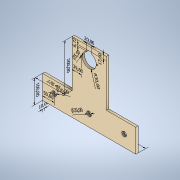
# Autodesk Inventor part: InnenUnten
Saved by Autodesk Inventor 2020.3 (Build 243373010, 373A)
## iProperties
Created: 2021-02-11
Part Number: InnenUnten
Material: Generisch
Document SubType Name: Modeling
Designer: Stefan
Density: 1 g/cm^3
Appearance: Pappel
Author: Stefan
Autodesk Inventor part; units mm, degrees
ref_plane "YZ Plane" through (0, 0, 0) normal (1, 0, 0) x (0, 1, 0)
ref_plane "XZ Plane" through (0, 0, 0) normal (0, 1, 0) x (-1, 0, 0)
ref_plane "XY Plane" through (0, 0, 0) normal (0, 0, 1) x (1, 0, 0)
sketch "Skizze1" plane through (0, 0, 0) normal (0, 0, 1) x (1, 0, 0)
  line L0 (147.1952, 0) -> (147.1952, 200)
  line L1 (147.1952, 200) -> (0, 200)
  line L2 (0, 200) -> (0, 0)
  line L3 (0, 0) -> (-24.1421, 0)
  line L4 (-24.1421, 0) -> (-126.4024, 0)
  line L5 (-126.4024, 0) -> (-126.4024, -100)
  line L6 (-126.4024, -100) -> (273.5976, -100)
  line L7 (273.5976, -100) -> (273.5976, 0)
  line L8 (273.5976, 0) -> (171.3373, 0)
  line L9 (171.3373, 0) -> (147.1952, 0)
  circle A0 centre (223.5976, -50) radius 10
  circle A1 centre (-76.4024, -50) radius 10
  circle A2 centre (73.5976, -50) radius 10
  dimension "d34" = 20
  dimension "d35" = 90
  dimension "d36" = 90
  dimension "d37" = 90
  dimension "d38" = 126.4024
  dimension "d39" = 273.5976
  dimension "d40" = 400
  dimension "d41" = 200
  dimension "d42" = 100
  dimension "d43" = 0
  dimension "d44" = 0
  dimension "d45" = 0
  dimension "d46" = 0
  dimension "d47" = 0
  dimension "d48" = 100
  dimension "d49" = 0
  dimension "d50" = 50
  dimension "d51" = 50
  dimension "d52" = 102.2603
  dimension "d53" = 102.2603
  dimension "d54" = 200
  dimension "d55" = 126.4024
  dimension "d56" = 0
  dimension "d57" = 126.4024
  dimension "d58" = 200
  dimension "d59" = 50
  dimension "d60" = 200
  dimension "d61" = 273.5976
  dimension "d62" = 0
  dimension "d63" = 273.5976
  dimension "d64" = 297.7397
  dimension "d65" = 297.7397
  dimension "d66" = 350
  dimension "d67" = 50
  dimension "d68" = 0
  dimension "d69" = 400
  dimension "d70" = 100
  dimension "d71" = 400
  constraints: 20 end point, 5 parallel, 3 centre point, 2 equal radius, 1 horizontal, 1 vertical
  measures "d34" diameter of A0
  measures "d35" angle of L7 L8
  measures "d36" angle of L7 L3
  measures "d37" angle of L7 L4
  measures "d38" distance between parallel lines of L0 L7
  measures "d39" distance between parallel lines of L2 L7
  measures "d40" distance between parallel lines of L5 L7
  measures "d41" distance between parallel lines of L1 L9
  measures "d42" distance between parallel lines of L6 L9
  measures "d43" distance from line of L7.end L8
  measures "d44" distance from line of L7.end L9
  measures "d45" distance from line of L7.end L3
  measures "d46" distance from line of L7.end L4
  measures "d47" distance from line of L8.start L7
  measures "d48" distance from line of L7.start L8
  measures "d49" distance from line of L6.end L7
  measures "d50" distance from line of A0.centre L7
  measures "d51" distance from line of A0.centre L8
  measures "d52" distance from line of L9.start L7
  measures "d53" distance from line of L8.end L7
  measures "d54" distance from line of L0.end L8
  measures "d55" distance from line of L1.start L7
  measures "d56" distance from line of L0.start L8
  measures "d57" distance from line of L9.end L7
  measures "d58" distance from line of A2.centre L7
  measures "d59" distance from line of A2.centre L8
  measures "d60" distance from line of L2.start L8
  measures "d61" distance from line of L1.end L7
  measures "d62" distance from line of L2.end L8
  measures "d63" distance from line of L3.start L7
  measures "d64" distance from line of L3.end L7
  measures "d65" distance from line of L4.start L7
  measures "d66" distance from line of A1.centre L7
  measures "d67" distance from line of A1.centre L8
  measures "d68" distance from line of L5.start L8
  measures "d69" distance from line of L4.end L7
  measures "d70" distance from line of L5.end L8
  measures "d71" distance from line of L6.start L7
extrude "Extrusion1" add sketch "Skizze1" along normal blind 10
sketch "Skizze2" plane through (0, 0, 10) normal (0, 0, 1) x (1, 0, 0)
  arc A0 (63.5977, 176.2843) -> (83.5977, 176.2843) centre (73.5977, 148) ccw
  line L0 (147.1952, 200) -> (0, 200) projected
  line L1 (147.1952, 0) -> (147.1952, 200) projected
  line L2 (63.5977, 183) -> (83.5977, 183)
  line L3 (83.5977, 183) -> (83.5977, 176.2843)
  line L4 (63.5977, 176.2843) -> (63.5977, 183)
  circle A1 centre (39.5977, 148) radius 2.75
  circle A2 centre (107.5977, 148) radius 2.75
  point P0 (0, 0)
  dimension "d72" = 60
  dimension "d73" = 52
  dimension "d74" = 73.5975
  dimension "d75" = 35
  dimension "d76" = 20
  dimension "d77" = 83.5975
  dimension "d78" = 5.5
  dimension "d79" = 5.5
  dimension "d80" = 52
  dimension "d81" = 68
  dimension "d82" = 0
  dimension "d83" = 39.5975
  constraints: 6 end point, 3 centre point, 2 point on circle, 1 horizontal, 1 parallel, 1 perpendicular
  measures "d72" diameter of A0
  measures "d73" distance from line of L0 A0.centre
  measures "d74" distance from line of L1 A0.centre
  measures "d75" distance from line of L2 A0.centre
  measures "d76" distance of L2.start L2.end
  measures "d77" distance between parallel lines of L1 L4
  measures "d78" diameter of A1
  measures "d79" diameter of A2
  measures "d80" distance from line of L0 A2.centre
  measures "d81" distance of A1.centre A2.centre
  measures "d82" vertical distance of A1.centre A2.centre
  measures "d83" distance from line of L1 A2.centre
extrude "Extrusion2" cut sketch "Skizze2" against normal through all
